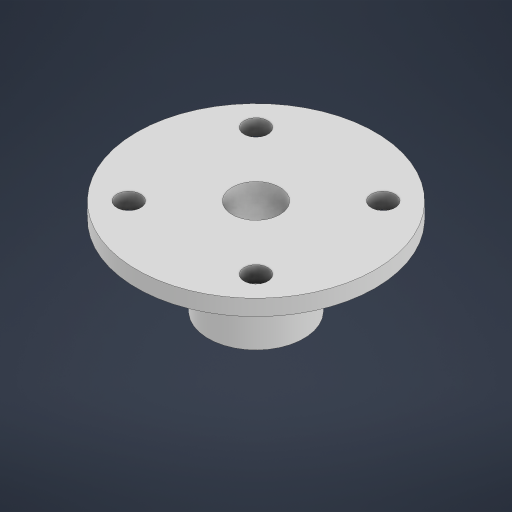
# Autodesk Inventor part: Flange
Saved by Autodesk Inventor 2023 (Build 270158000, 158)
## iProperties
Created: 2023-08-17
Part Number: Flange
Material: Generic
Document SubType Name: Modeling
Designer: Abhinav
Density: 1 g/cm^3
Appearance: Default
Author: Abhinav
Autodesk Inventor part; units mm, degrees
ref_plane "YZ Plane" through (0, 0, 0) normal (1, 0, 0) x (0, 1, 0)
ref_plane "XZ Plane" through (0, 0, 0) normal (0, 1, 0) x (-1, 0, 0)
ref_plane "XY Plane" through (0, 0, 0) normal (0, 0, 1) x (1, 0, 0)
sketch "Sketch1" plane through (0, 0, 0) normal (0, 1, 0) x (-1, 0, 0)
  circle A0 centre (0, 0) radius 3
  line L0 (-8, -8) -> (8, -8) construction
  line L1 (8, -8) -> (8, 8) construction
  line L2 (8, 8) -> (-8, 8) construction
  line L3 (-8, 8) -> (-8, -8) construction
  line L4 (-8, -8) -> (8, 8) construction
  line L5 (8, -8) -> (-8, 8) construction
  circle A1 centre (-8, 8) radius 1.5
  circle A2 centre (-8, -8) radius 1.5
  circle A3 centre (8, -8) radius 1.5
  circle A4 centre (8, 8) radius 1.5
  circle A5 centre (0, 0) radius 15
  circle A6 centre (0, 0) radius 6
  dimension "d8" = 6
  dimension "d9" = 16
  dimension "d11" = 3
  dimension "d12" = 30
  dimension "d15" = 12
  constraints: 12 end point, 7 centre point, 6 coincident, 3 equal radius, 2 midpoint, 2 parallel, 2 perpendicular, 1 horizontal, 4 other
  measures "d8" diameter of A0
  measures "d9" distance of L2.end L1.end
  measures "d11" diameter of A2
  measures "d12" diameter of A5
  measures "d15" diameter of A6
extrude "Extrusion1" add sketch "Sketch1" along normal blind 2 contours A5 | A6
extrude "Extrusion2" add sketch "Sketch1" against normal blind 10 contours A6
body "Solid1"
